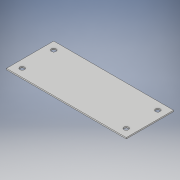
# Autodesk Inventor part: 76x30mm-PCB
Saved by Autodesk Inventor 2018 (Build 220112000, 112)
## iProperties
Created: 2018-04-09
Part Number: 76x30mm-PCB
Material: Generic
Document SubType Name: Modeling
Designer: bbramman
Density: 1 g/cm^3
Appearance: Default
Author: bbramman
Autodesk Inventor part; units mm, degrees
ref_plane "YZ Plane" through (0, 0, 0) normal (1, 0, 0) x (0, 1, 0)
ref_plane "XZ Plane" through (0, 0, 0) normal (0, 1, 0) x (-1, 0, 0)
ref_plane "XY Plane" through (0, 0, 0) normal (0, 0, 1) x (1, 0, 0)
sketch "Sketch1" plane through (0, 0, 0) normal (0, 1, 0) x (-1, 0, 0)
  line L0 (-38, 15) -> (38, 15)
  line L1 (38, 15) -> (38, -15)
  line L2 (38, -15) -> (-38, -15)
  line L3 (-38, -15) -> (-38, 15)
  line L4 (-38, 15) -> (38, -15) construction
  line L5 (38, 15) -> (-38, -15) construction
  point P0 (0, 0)
  dimension "d0" = 76
  dimension "d1" = 30
  constraints: 12 end point, 2 midpoint, 2 parallel, 1 horizontal, 1 perpendicular
  measures "d0" distance of L1.end L2.end
  measures "d1" distance of L0.end L1.end
extrude "Extrusion1" add sketch "Sketch1" along normal mid plane 0.7874
sketch "Sketch2" plane through (0, 0.3937, 0) normal (0, 1, 0) x (1, 0, 0)
  circle A0 centre (-33, -10) radius 1.5
  circle A1 centre (-33, 10) radius 1.5
  circle A2 centre (33, -10) radius 1.5
  circle A3 centre (33, 10) radius 1.5
  point P0 (0, 0)
  dimension "d4" = 3
  dimension "d5" = 3
  dimension "d6" = 3
  dimension "d7" = 3
  constraints: 4 centre point
  measures "d4" diameter of A0
  measures "d5" diameter of A1
  measures "d6" diameter of A2
  measures "d7" diameter of A3
extrude "Extrusion2" cut sketch "Sketch2" against normal through all
body "Solid1"
